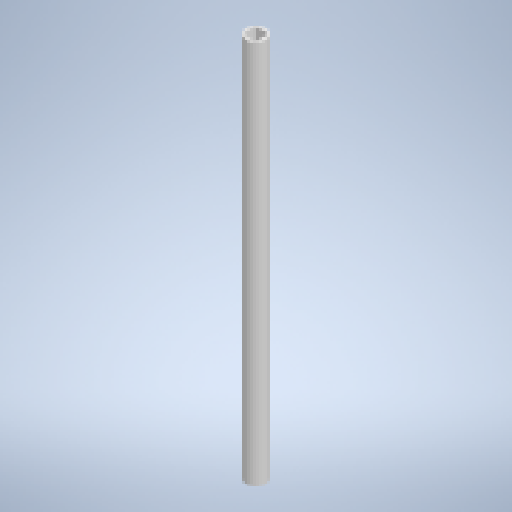
# Autodesk Inventor part: Separador largo
Saved by Autodesk Inventor 2024 (Build 280153000, 153)
## iProperties
Created: 2023-10-29
Part Number: Separador largo
Material: Genérico
Document SubType Name: Modeling
Designer: Soy_y
Density: 1 g/cm^3
Appearance: Valor por defecto
Author: Soy_y
Autodesk Inventor part; units mm, degrees
ref_plane "YZ Plane" through (0, 0, 0) normal (1, 0, 0) x (0, 1, 0)
ref_plane "XZ Plane" through (0, 0, 0) normal (0, 1, 0) x (-1, 0, 0)
ref_plane "XY Plane" through (0, 0, 0) normal (0, 0, 1) x (1, 0, 0)
sketch "Boceto1" plane through (0, 0, 0) normal (0, 1, 0) x (-1, 0, 0)
  line L0 (0.5, 0) -> (-0.375, 0)
  line L1 (0.125, 0.5) -> (0.125, 2.675)
  line L2 (-0.375, 3.175) -> (0.5, 3.175)
  line L3 (0, 2.675) -> (0, 0.5)
  circle A0 centre (3, 3) radius 5
  arc A1 (0.125, 2.675) -> (-0.375, 3.175) centre (-0.375, 2.675) ccw
  arc A2 (0, 0.5) -> (0.5, 0) centre (0.5, 0.5) ccw
  arc A3 (-0.375, 0) -> (0.125, 0.5) centre (-0.375, 0.5) ccw
  arc A4 (0.5, 3.175) -> (0, 2.675) centre (0.5, 2.675) ccw
  point P0 (0, 0)
  point P1 (0.125, 3.175)
  point P2 (0.125, 0)
  point P3 (0, 3.175)
  point P4 (0.0625, 2.9171)
  point P5 (0.0625, 0.2579)
  dimension "d0" = 0.125
  dimension "d1" = 3.175
  dimension "d4" = 10
  dimension "d5" = 0.5
  dimension "d6" = 0.5
  dimension "d7" = 0.5
  dimension "d8" = 0.5
  constraints: 8 end point, 8 point on circle, 8 point on line, 8 tangent, 5 centre point, 2 parallel, 1 horizontal, 1 perpendicular
  measures "d0" distance of point (0, 3.175) point (0.125, 3.175)
  measures "d1" distance of point (0.125, 0) point (0.125, 3.175)
  measures "d4" diameter of A0
  measures "d5" radius of A1
  measures "d6" radius of A2
  measures "d7" radius of A3
  measures "d8" radius of A4
extrude "Extrusión1" add sketch "Boceto1" along normal blind 190.5 contours A1 L2 A4 | A2 L3 A4 A1 L1 A3 | L0 A3 A2 | A0
